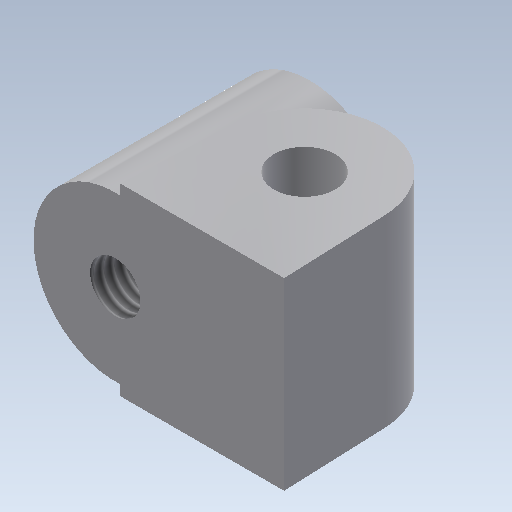
# Autodesk Inventor part: 500-171
Saved by Autodesk Inventor 2020 (Build 240168000, 168)
## iProperties
Created: 2015-04-18
Part Number: 500-171
Material: ABS Plastic
Document SubType Name: Modeling
Designer: Station9
Density: 1.06 g/cm^3
Appearance: Smooth - White
Mass: 0.821021 g
Surface Area: 6.54926 cm^2
Volume: 0.774548 cm^3
Author: Station9
Autodesk Inventor part; units mm, degrees
ref_plane "YZ Plane" through (0, 0, 0) normal (1, 0, 0) x (0, 1, 0)
ref_plane "XZ Plane" through (0, 0, 0) normal (0, 1, 0) x (-1, 0, 0)
ref_plane "XY Plane" through (0, 0, 0) normal (0, 0, 1) x (1, 0, 0)
sketch "Sketch1" plane through (0, 0, 0) normal (0, 1, 0) x (-1, 0, 0)
  line L0 (0, 0) -> (8, 0)
  line L1 (8, 0) -> (7.7971, -5.1496)
  line L2 (0.2029, -5.1496) -> (0, 0)
  arc A0 (0.2029, -5.1496) -> (7.7971, -5.1496) centre (4, -5) ccw
  line L3 (4, -5) -> (4, -1.2)
  dimension "d0" = 3.8
  dimension "d1" = 5
  dimension "d2" = 8
  constraints: 8 end point, 2 point on circle, 2 tangent, 1 centre point, 1 horizontal, 1 vertical, 1 other
  measures "d0" radius of A0
  measures "d1" distance from line of L0 L3.start
  measures "d2" distance of L0.start L0.end
extrude "Extrusion1" add sketch "Sketch1" along normal blind 9
sketch "Sketch2" plane through (-8, 0, 0) normal (0, 0, 1) x (1, 0, 0)
  line L0 (8, 0) -> (0, 0) projected
  line L1 (0, 0) -> (0, 9) projected
  circle A0 centre (-0.25, 4.5) radius 4
  line L2 (4, 0) -> (4, -1.6223)
  point P0 (0, 4.5)
  dimension "d5" = 8
  dimension "d6" = 4.25
  constraints: 2 end point, 2 midpoint, 1 centre point, 1 horizontal alignment, 1 vertical
  measures "d5" diameter of A0
  measures "d6" distance from line of A0.centre L2
extrude "Extrusion2" add sketch "Sketch2" against normal blind 9.5
hole "Hole1" at (-4, 9, -5) direction (0, -1, 0) diameter 3 depth 6
hole "Hole2" at (-8.25, 4.5, -9.5) direction (0, 0, 1) diameter 2.459 depth 12.05 thread size "M3x0.5" class "6H" standard "ISO Metric profile"
body "Solid1"
